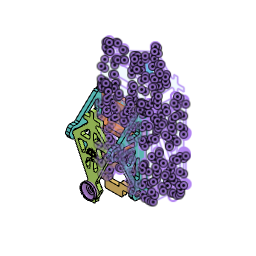
Katapult (Autodesk Fusion 360 design; units mm, degrees)
Autodesk Fusion 360 part; units mm, degrees
note: some values were not read from the file. Set by a fixed rule: which sketch regions a step uses.
(part 1 of 4)
sketch "Boden" plane through (0, 0, 0) normal (0, 1, 0) x (1, 0, 0)
  spline S0 degree 2 poles (146.3852, 44) (139.1926, 44) (132, 44) knots 58.903837 58.903837 58.903837 73.289058 73.289058 73.289058
  spline S1 degree 2 poles (132, 60) (138.2551, 60) (144.5102, 60) knots 21.966793 21.966793 21.966793 36.979059 36.979059 36.979059
  arc A0 (114.6662, 47.5529) -> (117.6148, 44) centre (117.6148, 47) ccw
  spline S2 degree 2 poles (119.4898, 60) (125.7449, 60) (132, 60) knots 109.599057 109.599057 109.599057 124.611322 124.611322 124.611322
  spline S3 degree 2 poles (147.4588, 57.5529) (148.3963, 52.5529) (149.3338, 47.5529) knots 41.135404 41.135404 41.135404 53.635404 53.635404 53.635404
  spline S4 degree 2 poles (132, 44) (124.8074, 44) (117.6148, 44) knots 73.289058 73.289058 73.289058 87.674279 87.674279 87.674279
  arc A1 (119.4898, 60) -> (116.5412, 57.5529) centre (119.4898, 57) ccw
  spline S5 degree 2 poles (114.6662, 47.5529) (115.6037, 52.5529) (116.5412, 57.5529) knots 92.942712 92.942712 92.942712 105.442712 105.442712 105.442712
  arc A2 (147.4588, 57.5529) -> (144.5102, 60) centre (144.5102, 57) ccw
  arc A3 (146.3852, 44) -> (149.3338, 47.5529) centre (146.3852, 47) ccw
  line L0 (157, 37.5) -> (157, 72.5)
  line L1 (107, 72.5) -> (107, 37.5)
  line L2 (157, 22.5) -> (162, 22.5)
  line L3 (162, 22.5) -> (162, 37.5)
  line L4 (162, 37.5) -> (157, 37.5)
  line L5 (157, 22.5) -> (157, 4)
  line L6 (157, 4) -> (107, 4)
  line L7 (107, 4) -> (107, 22.5)
  line L8 (107, 22.5) -> (102, 22.5)
  line L9 (102, 22.5) -> (102, 37.5)
  line L10 (102, 37.5) -> (107, 37.5)
  line L11 (107, 72.5) -> (102, 72.5)
  line L12 (102, 72.5) -> (102, 90.5)
  line L13 (157, 72.5) -> (162, 72.5)
  line L14 (162, 72.5) -> (162, 90.5)
  line L15 (120.5, 34) -> (143.5, 34)
  line L16 (143.5, 34) -> (143.5, 39)
  line L17 (143.5, 39) -> (120.5, 39)
  line L18 (120.5, 39) -> (120.5, 34)
  line L19 (102, 90.5) -> (107, 90.5)
  line L20 (107, 90.5) -> (107, 92)
  line L21 (157, 92) -> (157, 90.5)
  line L22 (157, 90.5) -> (162, 90.5)
  line L23 (107, 104) -> (107, 92)
  line L24 (107, 104) -> (117, 104)
  line L25 (117, 104) -> (117, 94)
  line L26 (117, 94) -> (132, 84.0491)
  line L27 (132, 84.0491) -> (147, 94)
  line L28 (147, 94) -> (147, 104)
  line L29 (147, 104) -> (156.9838, 104)
  line L30 (156.9838, 104) -> (157, 92)
  line L31 (114, 10) -> (127, 10)
  line L32 (127, 10) -> (114, 20)
  line L33 (114, 20) -> (114, 10)
  line L34 (150, 10) -> (137, 10)
  line L35 (137, 10) -> (150, 20)
  line L36 (150, 20) -> (150, 10)
  line L37 (127, 29) -> (127, 15)
  line L38 (127, 15) -> (109, 29)
  line L39 (109, 29) -> (127, 29)
  line L40 (137, 15) -> (155, 29)
  line L41 (155, 29) -> (137, 29)
  line L42 (137, 29) -> (137, 15)
  line L43 (129, 75) -> (129, 65)
  line L44 (129, 65) -> (115, 65)
  line L45 (115, 65) -> (115, 85)
  line L46 (115, 85) -> (129, 75)
  line L47 (135, 65) -> (149, 65)
  line L48 (149, 65) -> (149, 85)
  line L49 (149, 85) -> (135, 75)
  line L50 (135, 75) -> (135, 65)
  constraint horizontal L2
  constraint perpendicular L2 L3
  constraint perpendicular L2 L5
  constraint perpendicular L5 L6
  constraint parallel L6 L8
  constraint perpendicular L8 L9
  constraint perpendicular L1 L11
  constraint perpendicular L11 L12
  constraint perpendicular L0 L13
  constraint perpendicular L13 L14
  constraint horizontal L15
  constraint vertical L16
  constraint horizontal L17
  constraint vertical L18
  constraint perpendicular L12 L19
  constraint horizontal L22
  constraint perpendicular L23 L24
  constraint perpendicular L24 L25
  constraint parallel L25 L28
  constraint perpendicular L28 L29
  constraint horizontal L13
  constraint perpendicular L7 L31
  constraint perpendicular L31 L33
  constraint horizontal L34
  constraint perpendicular L34 L36
  constraint vertical L37
  constraint perpendicular L37 L39
  constraint horizontal L41
  constraint perpendicular L41 L42
  constraint parallel L42 L43
  constraint perpendicular L43 L44
  constraint perpendicular L44 L45
  constraint perpendicular L43 L47
  constraint perpendicular L47 L48
  constraint perpendicular L47 L50
sketch "Halter" plane through (0, 0, 0) normal (0, 1, 0) x (1, 0, 0)
  spline S0 degree 2 poles (99.3634, 51.0396) (99.5525, 51.4619) (99.5525, 51.9341) knots -102.762151 -102.762151 -102.762151 -101.834856 -101.834856 -101.834856 weights 1 0.973249 1
  spline S1 degree 2 poles (98.2087, 103.4619) (98.2087, 104.4619) (97.3128, 104.4619) knots -41.403496 -41.403496 -41.403496 -39.8327 -39.8327 -39.8327 weights 1 0.707107 1
  line L0 (83.4263, 70.9619) -> (83.4263, 63.4619)
  spline S2 degree 2 poles (93.7291, 43.4619) (93.7291, 42.4619) (94.6251, 42.4619) knots -116.78571 -116.78571 -116.78571 -115.214913 -115.214913 -115.214913 weights 1 0.707107 1
  spline S3 degree 2 poles (90.5935, 61.4619) (92.3853, 61.4619) (92.3853, 59.4619) knots -136.264428 -136.264428 -136.264428 -133.122835 -133.122835 -133.122835 weights 1 0.707107 1
  line L1 (83.4263, 75.9619) -> (83.4263, 70.9619)
  spline S4 degree 2 poles (83.4263, 63.4619) (83.4263, 61.4619) (85.2181, 61.4619) knots -145.40602 -145.40602 -145.40602 -142.264428 -142.264428 -142.264428 weights 1 0.707107 1
  spline S5 degree 2 poles (92.5745, 95.8842) (92.3853, 95.4619) (92.3853, 94.9898) knots -27.379937 -27.379937 -27.379937 -26.452642 -26.452642 -26.452642 weights 1 0.973249 1
  line L2 (94.6251, 42.4619) -> (97.3128, 42.4619)
  line L3 (93.7291, 103.4619) -> (93.7291, 98.4619)
  line L4 (97.7607, 66.4619) -> (94.1771, 66.4619)
  spline S6 degree 2 poles (92.3853, 51.9341) (92.3853, 51.4619) (92.5745, 51.0396) knots -125.594971 -125.594971 -125.594971 -124.667676 -124.667676 -124.667676 weights 1 0.973249 1
  line L5 (99.5525, 51.9341) -> (99.5525, 64.4619)
  spline S7 degree 2 poles (97.7607, 80.4619) (99.5525, 80.4619) (99.5525, 82.4619) knots -65.882214 -65.882214 -65.882214 -62.740621 -62.740621 -62.740621 weights 1 0.707107 1
  line L6 (93.7291, 48.4619) -> (93.7291, 43.4619)
  line L7 (99.5525, 82.4619) -> (99.5525, 94.9898)
  line L8 (94.1771, 80.4619) -> (97.7607, 80.4619)
  line L9 (94.1771, 73.4619) -> (94.1771, 80.4619)
  line L10 (93.7291, 98.4619) -> (92.5745, 95.8842)
  line L11 (94.1771, 66.4619) -> (94.1771, 73.4619)
  line L12 (98.2087, 98.4619) -> (98.2087, 103.4619)
  line L13 (92.3853, 59.4619) -> (92.3853, 51.9341)
  spline S8 degree 2 poles (92.3853, 87.4619) (92.3853, 85.4619) (90.5935, 85.4619) knots -18.924778 -18.924778 -18.924778 -15.783185 -15.783185 -15.783185 weights 1 0.707107 1
  line L14 (85.2181, 61.4619) -> (90.5935, 61.4619)
  spline S9 degree 2 poles (99.5525, 94.9898) (99.5525, 95.4619) (99.3634, 95.8842) knots -50.212757 -50.212757 -50.212757 -49.285462 -49.285462 -49.285462 weights 1 0.973249 1
  spline S10 degree 2 poles (99.5525, 64.4619) (99.5525, 66.4619) (97.7607, 66.4619) knots -89.306992 -89.306992 -89.306992 -86.165399 -86.165399 -86.165399 weights 1 0.707107 1
  line L15 (98.2087, 43.4619) -> (98.2087, 48.4619)
  line L16 (92.3853, 94.9898) -> (92.3853, 87.4619)
  spline S11 degree 2 poles (94.6251, 104.4619) (93.7291, 104.4619) (93.7291, 103.4619) knots -36.8327 -36.8327 -36.8327 -35.261903 -35.261903 -35.261903 weights 1 0.707107 1
  line L17 (92.5745, 51.0396) -> (93.7291, 48.4619)
  line L18 (83.4263, 83.4619) -> (83.4263, 75.9619)
  spline S12 degree 2 poles (85.2181, 85.4619) (83.4263, 85.4619) (83.4263, 83.4619) knots -9.783185 -9.783185 -9.783185 -6.641593 -6.641593 -6.641593 weights 1 0.707107 1
  line L19 (97.3128, 104.4619) -> (94.6251, 104.4619)
  line L20 (90.5935, 85.4619) -> (85.2181, 85.4619)
  spline S13 degree 2 poles (97.3128, 42.4619) (98.2087, 42.4619) (98.2087, 43.4619) knots -112.214913 -112.214913 -112.214913 -110.644117 -110.644117 -110.644117 weights 1 0.707107 1
  line L21 (99.3634, 95.8842) -> (98.2087, 98.4619)
  line L22 (98.2087, 48.4619) -> (99.3634, 51.0396)
sketch "Seiten" plane through (0, 0, 0) normal (0, 1, 0) x (1, 0, 0)
  spline S0 degree 2 poles (8, 106) (5.5, 106) (3, 106) knots -333.29607 -333.29607 -333.29607 -328.29607 -328.29607 -328.29607
  line L0 (0, 42) -> (0, 41)
  line L1 (11.4183, 106) -> (8, 106)
  arc A0 (1, 43) -> (3, 45) centre (1, 45) ccw
  line L2 (38.5159, 82.0817) -> (14.1539, 104.9183)
  arc A1 (14.1539, 104.9183) -> (11.4183, 106) centre (11.4183, 102) ccw
  line L3 (3, 66) -> (3, 45)
  arc A2 (1, 43) -> (0, 42) centre (1, 42) ccw
  arc A3 (3, 66) -> (1, 68) centre (1, 66) ccw
  arc A4 (0, 69) -> (1, 68) centre (1, 69) ccw
  line L4 (0, 103) -> (0, 69)
  arc A5 (3, 106) -> (0, 103) centre (3, 103) ccw
  arc A6 (49.4848, 79) -> (46.0207, 81) centre (46.0207, 77) ccw
  arc A7 (38.5159, 82.0817) -> (41.2515, 81) centre (41.2515, 85) ccw
  line L5 (42.2092, 66) -> (46.0207, 66)
  arc A8 (18.9309, 21.8917) -> (19.0866, 18.1897) centre (22.5507, 20.1897) ccw
  circle A9 centre (14, 13) radius 3.5355
  line L6 (18.9309, 21.8917) -> (38.5894, 63.702)
  arc A10 (20.9282, 11) -> (20.9282, 15) centre (17.4641, 13) ccw
  arc A11 (42.2092, 66) -> (38.5894, 63.702) centre (42.2092, 62) ccw
  line L7 (20.9282, 15) -> (19.0866, 18.1897)
  line L8 (51.5056, 75.5) -> (49.4848, 79)
  circle A12 centre (44, 73.5) radius 3.5355
  line L9 (49.4848, 68) -> (51.5056, 71.5)
  line L10 (9.9585, 6) -> (15.7321, 6)
  arc A13 (51.5056, 71.5) -> (51.5056, 75.5) centre (48.0415, 73.5) ccw
  arc A14 (0, 9) -> (3, 6) centre (3, 9) ccw
  line L11 (19.1962, 8) -> (20.9282, 11)
  arc A15 (15.7321, 6) -> (19.1962, 8) centre (15.7321, 10) ccw
  line L12 (46.0207, 81) -> (41.2515, 81)
  line L13 (0, 41) -> (0, 9)
  line L14 (3, 6) -> (9.9585, 6)
  arc A16 (46.0207, 66) -> (49.4848, 68) centre (46.0207, 70) ccw
  line L15 (18.5, 71) -> (33.5, 71)
  line L16 (33.5, 71) -> (33.5, 76)
  line L17 (33.5, 76) -> (18.5, 76)
  line L18 (18.5, 76) -> (18.5, 71)
  line L19 (3, 72.5) -> (8, 72.5)
  line L20 (8, 72.5) -> (8, 87.5)
  line L21 (8, 87.5) -> (3, 87.5)
  line L22 (3, 87.5) -> (3, 72.5)
  line L23 (3, 19.5) -> (8, 19.5)
  line L24 (8, 19.5) -> (8, 37.5)
  line L25 (8, 37.5) -> (3, 37.5)
  line L26 (3, 37.5) -> (3, 19.5)
  line L27 (12, 20) -> (12, 62)
  line L28 (12, 62) -> (23, 43)
  line L29 (23, 43) -> (12, 20)
  line L30 (34, 66) -> (26, 48)
  line L31 (26, 48) -> (15.5, 66)
  line L32 (15.5, 66) -> (34, 66)
  line L33 (12, 81) -> (32.5, 81)
  line L34 (32.5, 81) -> (12, 100)
  line L35 (12, 100) -> (12, 81)
  dimension "d27" = 15
  constraint horizontal L15
  constraint vertical L16
  constraint horizontal L17
  constraint vertical L18
  constraint horizontal L19
  constraint vertical L20
  constraint horizontal L21
  constraint vertical L22
  constraint horizontal L23
  constraint vertical L24
  constraint horizontal L25
  constraint vertical L26
  constraint vertical L27
  constraint horizontal L32
  constraint horizontal L33
  constraint perpendicular L33 L35
  measures "d27" distance of L16.end L17.end
sketch "Hebel" plane through (0, 0, 0) normal (0, 1, 0) x (1, 0, 0)
  line L0 (73.128, 41.6803) -> (76.7542, 51.7057)
  spline S0 degree 2 poles (42, 34) (51.4199, 25.1097) (60.8397, 16.2193) (61.8269, 15.2877) (61.3256, 14.0262) (60.8244, 12.7648) (59.467, 12.7648) (58.2335, 12.7648) (57, 12.7648) (56, 12.7648) (56, 11.7648) (56, 10.2648) (56, 8.7648) (56, 7.7648) (57, 7.7648) (59.75, 7.7648) (62.5, 7.7648) (64.5, 7.7648) (64.5, 5.7648) (64.5, 3.0148) (64.5, 0.2648) (64.5, -0.7352) (65.5, -0.7352) (67, -0.7352) (68.5, -0.7352) (69.5, -0.7352) (69.5, 0.2648) (69.5, 3.0148) (69.5, 5.7648) (69.5, 7.7648) (71.5, 7.7648) (74.25, 7.7648) (77, 7.7648) (78, 7.7648) (78, 8.7648) (78, 10.2648) (78, 11.7648) (78, 12.7648) (77, 12.7648) (75.7665, 12.7648) (74.533, 12.7648) (73.1756, 12.7648) (72.6744, 14.0262) (72.1731, 15.2877) (73.1603, 16.2193) (82.5801, 25.1097) (92, 34) knots -180.29335 -180.29335 -180.29335 -154.387975 -154.387975 -152.002869 -152.002869 -149.617763 -149.617763 -147.150765 -147.150765 -145.579969 -145.579969 -142.579969 -142.579969 -141.009172 -141.009172 -135.509172 -135.509172 -132.36758 -132.36758 -126.86758 -126.86758 -125.296783 -125.296783 -122.296783 -122.296783 -120.725987 -120.725987 -115.225987 -115.225987 -112.084394 -112.084394 -106.584394 -106.584394 -105.013598 -105.013598 -102.013598 -102.013598 -100.442802 -100.442802 -97.975804 -97.975804 -95.590698 -95.590698 -93.205592 -93.205592 -67.300216 -67.300216 -67.300216 weights 1 1 1 0.827432 1 0.827432 1 1 1 0.707107 1 1 1 0.707107 1 1 1 0.707107 1 1 1 0.707107 1 1 1 0.707107 1 1 1 0.707107 1 1 1 0.707107 1 1 1 0.707107 1 1 1 0.827432 1 0.827432 1 1 1
  arc A0 (83.3325, 39) -> (85.1436, 41.8486) centre (83.3325, 41) ccw
  arc A1 (75.1144, 61.8724) -> (75.0447, 63.4012) centre (73.2337, 62.5527) ccw
  line L1 (71.5, 34) -> (79.6823, 34)
  line L2 (81.055, 30.5455) -> (72.8727, 22.8232)
  line L3 (69.5, 24.2777) -> (69.5, 32)
  arc A2 (73.311, 67.1012) -> (69.5, 66.2526) centre (71.5, 66.2526) ccw
  line L4 (69.5, 66.2526) -> (69.5, 57.7595)
  arc A3 (80.446, 51.8741) -> (76.7542, 51.7057) centre (78.6349, 51.0255) ccw
  line L5 (80.446, 51.8741) -> (85.1436, 41.8486)
  arc A4 (61.1273, 22.8232) -> (64.5, 24.2777) centre (62.5, 24.2777) ccw
  line L6 (64.5, 24.2777) -> (64.5, 32)
  arc A5 (54.3177, 34) -> (52.945, 30.5455) centre (54.3177, 32) ccw
  line L7 (52.945, 30.5455) -> (61.1273, 22.8232)
  arc A6 (48.8564, 41.8486) -> (50.6675, 39) centre (50.6675, 41) ccw
  line L8 (50.6675, 39) -> (58.9913, 39)
  arc A7 (71.5, 34) -> (69.5, 32) centre (71.5, 32) ccw
  line L9 (62.5, 34) -> (54.3177, 34)
  arc A8 (69.5, 24.2777) -> (72.8727, 22.8232) centre (71.5, 24.2777) ccw
  line L10 (73.3808, 57.0792) -> (75.1144, 61.8724)
  arc A9 (60.6192, 57.0792) -> (64.5, 57.7595) centre (62.5, 57.7595) ccw
  line L11 (60.6192, 57.0792) -> (58.8856, 61.8724)
  line L12 (83.3325, 39) -> (75.0087, 39)
  arc A10 (73.128, 41.6803) -> (75.0087, 39) centre (75.0087, 41) ccw
  arc A11 (69.5, 57.7595) -> (73.3808, 57.0792) centre (71.5, 57.7595) ccw
  arc A12 (64.5, 32) -> (62.5, 34) centre (62.5, 32) ccw
  line L13 (60.872, 41.6803) -> (57.2458, 51.7057)
  arc A13 (58.9913, 39) -> (60.872, 41.6803) centre (58.9913, 41) ccw
  line L14 (58.9553, 63.4012) -> (60.689, 67.1012)
  arc A14 (64.5, 66.2526) -> (60.689, 67.1012) centre (62.5, 66.2526) ccw
  line L15 (64.5, 66.2526) -> (64.5, 57.7595)
  arc A15 (57.2458, 51.7057) -> (53.554, 51.8741) centre (55.3651, 51.0255) ccw
  arc A16 (81.055, 30.5455) -> (79.6823, 34) centre (79.6823, 32) ccw
  arc A17 (58.9553, 63.4012) -> (58.8856, 61.8724) centre (60.7663, 62.5527) ccw
  line L16 (53.554, 51.8741) -> (48.8564, 41.8486)
  line L17 (75.0447, 63.4012) -> (73.311, 67.1012)
  spline S1 degree 2 poles (98, 38) (98, 39) (97, 39) (94.5, 39) (92, 39) knots -57.72942 -57.72942 -57.72942 -56.158624 -56.158624 -51.158624 -51.158624 -51.158624 weights 1 0.707107 1 1 1
  spline S2 degree 2 poles (92, 34) (94.5, 34) (97, 34) (98, 34) (98, 35) knots -67.300216 -67.300216 -67.300216 -62.300216 -62.300216 -60.72942 -60.72942 -60.72942 weights 1 1 1 0.707107 1
  line L18 (98, 35) -> (98, 38)
  line L19 (36, 37.9531) -> (36, 38)
  spline S3 degree 2 poles (36, 35) (36, 34) (37, 34) (39.5, 34) (42, 34) knots -186.864147 -186.864147 -186.864147 -185.29335 -185.29335 -180.29335 -180.29335 -180.29335 weights 1 0.707107 1 1 1
  spline S4 degree 2 poles (42, 39) (39.5, 39) (37, 39) (36, 39) (36, 38) (36, 37.9766) (36, 37.9531) knots -196.434943 -196.434943 -196.434943 -191.434943 -191.434943 -189.864147 -189.864147 -189.817295 -189.817295 -189.817295 weights 1 1 1 0.707107 1 1 1
  line L20 (36, 35) -> (36, 37.9531)
  circle A18 centre (67, 90.2648) radius 0.375
  line L21 (72.1962, 102.2483) -> (72.1962, 103.0296)
  line L22 (69.4512, 105.0296) -> (70.1962, 105.0296)
  line L23 (67, 105.0296) -> (62, 105.0296)
  line L24 (62, 105.0296) -> (62, 100)
  line L25 (62, 100) -> (56.5, 90)
  line L26 (56.5, 90) -> (62, 81)
  line L27 (62, 81) -> (42, 39)
  line L28 (67, 105.0296) -> (72, 105.0296)
  line L29 (72, 105.0296) -> (72, 100)
  line L30 (72, 100) -> (77.5, 90)
  line L31 (77.5, 90) -> (72, 81)
  line L32 (72, 81) -> (92, 39)
  dimension "d48" = 0.75
  constraint coincident L19.end S4
  constraint vertical L19
  constraint vertical L21
  constraint perpendicular L21 L22
  constraint horizontal L23
  constraint perpendicular L23 L24
  constraint perpendicular L23 L29
  measures "d48" diameter of A18
sketch "Quer" plane through (0, 0, 0) normal (0, 1, 0) x (1, 0, 0)
  line L0 (163.6644, 44.088) -> (163.6644, 30.588)
  line L1 (163.6644, 80.588) -> (163.6644, 67.088)
  line L2 (163.6644, 67.088) -> (158.6644, 67.088)
  line L3 (158.6644, 44.088) -> (163.6644, 44.088)
  line L4 (163.6644, 30.588) -> (174.1644, 30.588)
  line L5 (174.1644, 80.588) -> (163.6644, 80.588)
  line L6 (174.1644, 85.588) -> (174.1644, 80.588)
  arc A0 (175.8002, 69.9888) -> (174.6644, 67.6383) centre (177.6644, 67.6383) ccw
  line L7 (189.1644, 85.588) -> (174.1644, 85.588)
  line L8 (189.1644, 80.588) -> (189.1644, 85.588)
  line L9 (174.6644, 55.588) -> (174.6644, 67.6383)
  line L10 (174.1644, 30.588) -> (174.1644, 25.588)
  line L11 (189.1644, 25.588) -> (189.1644, 30.588)
  line L12 (174.6644, 43.5376) -> (174.6644, 55.588)
  arc A1 (174.6644, 43.5376) -> (175.8002, 41.1871) centre (177.6644, 43.5376) ccw
  line L13 (174.1644, 25.588) -> (189.1644, 25.588)
  line L14 (158.6644, 67.088) -> (158.6644, 44.088)
  line L15 (189.1644, 30.588) -> (191, 30.588)
  line L16 (191, 30.588) -> (191, 32)
  line L17 (191, 32) -> (175.8002, 41.1871)
  line L18 (189.1644, 80.588) -> (191, 80.588)
  line L19 (191, 80.588) -> (191, 79)
  line L20 (191, 79) -> (175.8002, 69.9888)
  constraint perpendicular L11 L15
  constraint perpendicular L15 L16
  constraint perpendicular L16 L18
  constraint perpendicular L15 L19
sketch "makerhafen-logo" plane through (78.9239, 0, 23.4593) normal (0, 1, 0) x (1, 0, 0)
  line L0 (3.0435, 0.3482) -> (3.0389, 0.4531)
  line L1 (3.0389, 0.4531) -> (3.0716, 0.553)
  line L2 (2.5336, 2.4375) -> (2.6594, 2.4375)
  line L3 (3.8976, 2.125) -> (3.8976, 2.0272)
  line L4 (3.3321, 2.1809) -> (3.3321, 2.0276)
  line L5 (1.114, 2.2681) -> (1.2274, 2.4375)
  line L6 (1.2274, 2.4375) -> (1.3404, 2.4375)
  line L7 (1.3404, 2.4375) -> (1.237, 2.2876)
  line L8 (1.237, 2.2876) -> (1.3653, 2.0276)
  line L9 (3.8536, 1.161) -> (3.855, 1.1648)
  line L10 (3.8701, 1.2062) -> (3.8445, 1.2134)
  line L11 (3.773, 1.2543) -> (3.7021, 1.3317)
  line L12 (0, 2.4375) -> (0.1643, 2.4375)
  line L13 (0.1643, 2.4375) -> (0.2237, 2.2199)
  line L14 (0.2237, 2.2199) -> (0.2804, 2.4375)
  line L15 (0.2804, 2.4375) -> (0.4453, 2.4375)
  line L16 (0.0938, 2.0276) -> (0, 2.0276)
  line L17 (0, 2.0276) -> (0, 2.4375)
  line L18 (3.8445, 1.2134) -> (3.773, 1.2543)
  line L19 (2.4219, 0.1221) -> (2.4498, 0.0447)
  line L20 (2.4498, 0.0447) -> (2.4525, 0.0182)
  line L21 (2.4525, 0.0182) -> (2.4564, 0.0189)
  line L22 (3.7483, 1.1867) -> (3.8294, 1.172)
  line L23 (3.855, 1.1648) -> (3.8688, 1.2024)
  line L24 (3.6442, 1.1731) -> (3.7483, 1.1867)
  line L25 (3.6571, 1.5112) -> (3.6617, 1.5374)
  line L26 (3.5413, 0.6742) -> (3.4882, 0.7372)
  line L27 (3.0719, 0.2709) -> (3.0435, 0.3482)
  line L28 (3.087, 0.2489) -> (3.0719, 0.2709)
  line L29 (3.4414, 0.6821) -> (3.5126, 0.6406)
  line L30 (3.4481, 0.8343) -> (3.4449, 0.9392)
  line L31 (3.1608, 0.654) -> (3.2349, 0.6899)
  line L32 (3.0389, 0.4531) -> (3.0716, 0.553)
  line L33 (2.3853, 3.8451) -> (2.3988, 3.8779)
  line L34 (2.3988, 3.8779) -> (2.4006, 3.8841)
  line L35 (1.6118, 0.4999) -> (1.4882, 0.5595)
  line L36 (3.2349, 0.6899) -> (3.3389, 0.7049)
  line L37 (3.5126, 0.6406) -> (3.5317, 0.622)
  line L38 (3.5603, 0.6555) -> (3.5629, 0.6586)
  line L39 (3.5516, 1.1236) -> (3.6442, 1.1731)
  line L40 (3.4676, 1.0185) -> (3.4809, 1.0414)
  line L41 (3.3389, 0.7049) -> (3.4414, 0.6821)
  line L42 (3.1404, 0.6368) -> (3.1608, 0.654)
  line L43 (3.4882, 0.7372) -> (3.4481, 0.8343)
  line L44 (1.7416, 0.4524) -> (1.6118, 0.4999)
  line L45 (3.12, 0.6197) -> (3.1404, 0.6368)
  line L46 (3.0716, 0.553) -> (3.12, 0.6197)
  line L47 (3.5629, 0.6586) -> (3.5413, 0.6742)
  line L48 (3.0435, 0.3482) -> (3.0389, 0.4531)
  line L49 (3.4809, 1.0414) -> (3.4942, 1.0645)
  line L50 (3.5343, 0.625) -> (3.5603, 0.6555)
  line L51 (3.5317, 0.622) -> (3.5343, 0.625)
  line L52 (2.2074, 2.3253) -> (2.2071, 2.3169)
  line L53 (2.2071, 2.3169) -> (2.2072, 2.3115)
  line L54 (2.2072, 2.3115) -> (2.1951, 2.2592)
  line L55 (3.7128, 2.343) -> (3.7128, 2.2835)
  line L56 (2.1927, 2.2544) -> (2.1903, 2.2499)
  line L57 (2.1951, 2.2592) -> (2.1927, 2.2544)
  line L58 (1.4324, 0.369) -> (1.5352, 0.3905)
  line L59 (0.9862, 0.7052) -> (1.0901, 0.6902)
  line L60 (2.358, 0.2054) -> (2.4219, 0.1221)
  line L61 (2.4998, 0.0265) -> (2.4932, 0.0523)
  line L62 (0.7626, 0.6593) -> (0.7651, 0.6562)
  line L63 (1.9666, 0.2054) -> (2.0558, 0.2607)
  line L64 (0.3556, 1.8261) -> (0.3556, 1.8201)
  line L65 (1.6171, 0.382) -> (1.6422, 0.3729)
  line L66 (1.3437, 0.3126) -> (1.4324, 0.369)
  line L67 (2.3434, 1.1709) -> (2.3441, 1.1666)
  line L68 (2.3441, 1.1666) -> (2.3953, 0.9132)
  line L69 (2.3953, 0.9132) -> (2.3955, 0.9124)
  line L70 (2.3955, 0.9124) -> (2.3964, 0.9052)
  line L71 (1.6422, 0.3729) -> (1.6672, 0.3638)
  line L72 (2.0687, 1.6326) -> (2.0687, 1.604)
  line L73 (2.0687, 1.604) -> (2.0684, 1.6011)
  line L74 (2.0684, 1.6011) -> (2.0676, 1.596)
  line L75 (3.5126, 0.6406) -> (3.5317, 0.622)
  line L76 (3.5317, 0.622) -> (3.5343, 0.625)
  line L77 (2.5894, 0.3175) -> (2.6576, 0.3637)
  line L78 (1.0901, 0.6902) -> (1.1642, 0.6542)
  line L79 (2.9769, 2.1084) -> (2.8671, 2.1084)
  line L80 (2.0236, 2.2719) -> (2.027, 2.2717)
  line L81 (1.8443, 2.4375) -> (2.058, 2.4375)
  line L82 (2.4525, 0.0182) -> (2.4564, 0.0189)
  line L83 (2.4498, 0.0447) -> (2.4525, 0.0182)
  line L84 (2.4958, 0.0258) -> (2.4998, 0.0265)
  line L85 (2.3964, 0.9052) -> (2.3964, 0.9028)
  line L86 (2.3964, 0.9028) -> (2.4026, 0.9061)
  line L87 (2.4026, 0.9061) -> (2.4176, 0.9228)
  line L88 (2.4176, 0.9228) -> (2.438, 0.9563)
  line L89 (0.8373, 0.7378) -> (0.7842, 0.6749)
  line L90 (0.6599, 1.5643) -> (0.6646, 1.5381)
  line L91 (0.3556, 1.8066) -> (0.3556, 1.8021)
  line L92 (2.8925, 0.3688) -> (2.9811, 0.3122)
  line L93 (0.7651, 0.6562) -> (0.7907, 0.6255)
  line L94 (3.0488, 0.2268) -> (3.0834, 0.2468)
  line L95 (1.7354, 0.3175) -> (1.8003, 0.2349)
  line L96 (3.3802, 1.8021) -> (3.3802, 1.8081)
  line L97 (0.7933, 0.6225) -> (0.8124, 0.6411)
  line L98 (0.8124, 0.6411) -> (0.8836, 0.6825)
  line L99 (2.4564, 0.0189) -> (2.4958, 0.0258)
  line L100 (3.0337, 0.2489) -> (3.0453, 0.2249)
  line L101 (1.8249, 0.0265) -> (1.8288, 0.0258)
  line L102 (2.5245, 0.2349) -> (2.5894, 0.3175)
  line L103 (2.4932, 0.0523) -> (2.4928, 0.1347)
  line L104 (1.2795, 0.2252) -> (1.291, 0.2492)
  line L105 (3.5343, 0.625) -> (3.5603, 0.6555)
  line L106 (3.5603, 0.6555) -> (3.5629, 0.6586)
  line L107 (3.5629, 0.6586) -> (3.5413, 0.6742)
  line L108 (2.0676, 1.596) -> (2.0534, 1.5462)
  line L109 (2.0534, 1.5462) -> (2.0514, 1.5414)
  line L110 (2.0514, 1.5414) -> (2.0497, 1.5367)
  line L111 (2.9811, 0.3122) -> (3.0337, 0.2489)
  line L112 (0.3556, 1.783) -> (0.3556, 1.7787)
  line L113 (1.2813, 0.3485) -> (1.2528, 0.2712)
  line L114 (2.4928, 0.1347) -> (2.5245, 0.2349)
  line L115 (3.0716, 0.553) -> (3.12, 0.6197)
  line L116 (3.12, 0.6197) -> (3.1404, 0.6368)
  line L117 (3.1404, 0.6368) -> (3.1608, 0.654)
  line L118 (2.3255, 1.1962) -> (2.3376, 1.1836)
  line L119 (2.3376, 1.1836) -> (2.3434, 1.1709)
  line L120 (1.9026, 0.1221) -> (1.9666, 0.2054)
  line L121 (2.7077, 0.3819) -> (2.7896, 0.3903)
  line L122 (1.2859, 0.4534) -> (1.2813, 0.3485)
  line L123 (1.2378, 0.2492) -> (1.2412, 0.2471)
  line L124 (2.6827, 0.3728) -> (2.7077, 0.3819)
  line L125 (2.6576, 0.3637) -> (2.6827, 0.3728)
  line L126 (1.8315, 0.0523) -> (1.8249, 0.0265)
  line L127 (2.438, 0.9563) -> (2.4559, 0.9966)
  line L128 (2.4559, 0.9966) -> (2.4665, 1.0268)
  line L129 (1.1846, 0.637) -> (1.2049, 0.62)
  line L130 (1.8003, 0.2349) -> (1.8318, 0.1347)
  line L131 (2.1356, 0.2808) -> (2.1623, 0.2808)
  line L132 (1.2049, 0.62) -> (1.2532, 0.5532)
  line L133 (1.8721, 0.0182) -> (1.8747, 0.0447)
  line L134 (1.9786, 1.3712) -> (1.9629, 1.3493)
  line L135 (1.9629, 1.3493) -> (1.9461, 1.33)
  line L136 (1.9461, 1.33) -> (1.9287, 1.3096)
  line L137 (0.8776, 0.8348) -> (0.8373, 0.7378)
  line L138 (2.0385, 1.5022) -> (2.0354, 1.4931)
  line L139 (2.0354, 1.4931) -> (2.0344, 1.49)
  line L140 (2.0344, 1.49) -> (2.031, 1.4804)
  line L141 (2.2687, 0.2607) -> (2.358, 0.2054)
  line L142 (3.1608, 0.654) -> (3.2349, 0.6899)
  line L143 (3.2349, 0.6899) -> (3.3389, 0.7049)
  line L144 (3.3389, 0.7049) -> (3.4414, 0.6821)
  line L145 (3.4414, 0.6821) -> (3.5126, 0.6406)
  line L146 (2.031, 1.4804) -> (1.9884, 1.3877)
  line L147 (1.9884, 1.3877) -> (1.9832, 1.3789)
  line L148 (1.9832, 1.3789) -> (1.9786, 1.3712)
  line L149 (1.2759, 0.2272) -> (1.2795, 0.2252)
  line L150 (2.7896, 0.3903) -> (2.8925, 0.3688)
  line L151 (0.845, 1.042) -> (0.8583, 1.019)
  line L152 (3.0834, 0.2468) -> (3.087, 0.2489)
  line L153 (1.8681, 0.0189) -> (1.8721, 0.0182)
  line L154 (2.1623, 0.2808) -> (2.1889, 0.2808)
  line L155 (2.0497, 1.5367) -> (2.0449, 1.5225)
  line L156 (2.0449, 1.5225) -> (2.0413, 1.5112)
  line L157 (2.0413, 1.5112) -> (2.0385, 1.5022)
  line L158 (4.0936, 2.2258) -> (4.0936, 2.0278)
  line L159 (2.058, 2.4375) -> (2.0737, 2.4375)
  line L160 (0.4964, 1.1729) -> (0.5775, 1.1875)
  line L161 (0.845, 1.042) -> (0.8583, 1.019)
  line L162 (0.6631, 1.4297) -> (0.6239, 1.3323)
  line L163 (0.5528, 1.2549) -> (0.4813, 1.214)
  line L164 (0.7651, 0.6562) -> (0.7907, 0.6255)
  line L165 (1.97, 2.0276) -> (1.8443, 2.0276)
  line L166 (1.8443, 2.0276) -> (1.8443, 2.4375)
  line L167 (1.7507, 2.343) -> (1.5659, 2.343)
  line L168 (1.5659, 2.343) -> (1.5659, 2.2835)
  line L169 (0.4722, 1.1619) -> (0.4964, 1.1729)
  line L170 (0.7743, 1.1242) -> (0.8317, 1.0651)
  line L171 (0.4813, 1.214) -> (0.4557, 1.2069)
  line L172 (0.7933, 0.6225) -> (0.8124, 0.6411)
  line L173 (3.4481, 0.8343) -> (3.4449, 0.9392)
  line L174 (3.4449, 0.9392) -> (3.4676, 1.0185)
  line L175 (3.4676, 1.0185) -> (3.4809, 1.0414)
  line L176 (0.5564, 1.7179) -> (0.6264, 1.6395)
  line L177 (0.3822, 1.7807) -> (0.4633, 1.7665)
  line L178 (0.8124, 0.6411) -> (0.8836, 0.6825)
  line L179 (2.1889, 0.2808) -> (2.2687, 0.2607)
  line L180 (2.2687, 0.2607) -> (2.358, 0.2054)
  line L181 (2.358, 0.2054) -> (2.4219, 0.1221)
  line L182 (0.7907, 0.6255) -> (0.7933, 0.6225)
  line L183 (1.5631, 3.3276) -> (1.5675, 3.3102)
  line L184 (1.5675, 3.3102) -> (1.5796, 3.2908)
  line L185 (1.5796, 3.2909) -> (1.5978, 3.2772)
  line L186 (1.5978, 3.2772) -> (1.6147, 3.2713)
  line L187 (1.6147, 3.2713) -> (1.6205, 3.2708)
  line L188 (0.7626, 0.6593) -> (0.7651, 0.6562)
  line L189 (3.5413, 0.6742) -> (3.4882, 0.7372)
  line L190 (3.4882, 0.7372) -> (3.4481, 0.8343)
  line L191 (0.6816, 1.1738) -> (0.7743, 1.1242)
  line L192 (0.6691, 1.5119) -> (0.6631, 1.4297)
  line L193 (0.9862, 0.7052) -> (1.0901, 0.6902)
  line L194 (2.3927, 4.0582) -> (2.3613, 4.1039)
  line L195 (2.3613, 4.1039) -> (2.3176, 4.138)
  line L196 (2.3176, 4.138) -> (2.2782, 4.1549)
  line L197 (2.4109, 3.9939) -> (2.4092, 4.0038)
  line L198 (2.4092, 4.0038) -> (2.4072, 4.0177)
  line L199 (2.4072, 4.0177) -> (2.3927, 4.0582)
  line L200 (1.0901, 0.6902) -> (1.1642, 0.6542)
  line L201 (0.8317, 1.0651) -> (0.845, 1.042)
  line L202 (0.3556, 1.7787) -> (0.3822, 1.7807)
  line L203 (0.3556, 1.7962) -> (0.3556, 1.783)
  line L204 (0.8776, 0.8348) -> (0.8373, 0.7378)
  line L205 (0.4633, 1.7665) -> (0.5564, 1.7179)
  line L206 (0.8836, 0.6825) -> (0.9862, 0.7052)
  line L207 (0.8373, 0.7378) -> (0.7842, 0.6749)
  line L208 (1.1846, 0.637) -> (1.2049, 0.62)
  line L209 (0.8809, 0.9398) -> (0.8776, 0.8348)
  line L210 (1.6205, 3.2708) -> (1.6205, 3.4167)
  line L211 (1.6205, 3.4167) -> (1.6309, 3.4167)
  line L212 (0.5775, 1.1875) -> (0.6816, 1.1738)
  line L213 (0.6264, 1.6395) -> (0.6599, 1.5643)
  line L214 (0.8583, 1.019) -> (0.8809, 0.9398)
  line L215 (0.6239, 1.3323) -> (0.5528, 1.2549)
  line L216 (0.7842, 0.6749) -> (0.7626, 0.6593)
  line L217 (1.2049, 0.62) -> (1.2532, 0.5532)
  line L218 (1.1642, 0.6542) -> (1.1846, 0.637)
  line L219 (1.5659, 2.2835) -> (1.7153, 2.2835)
  line L220 (1.7153, 2.2835) -> (1.7153, 2.1926)
  line L221 (2.1623, 0.2808) -> (2.1889, 0.2808)
  line L222 (3.4809, 1.0414) -> (3.4942, 1.0645)
  line L223 (3.4942, 1.0645) -> (3.5516, 1.1236)
  line L224 (3.5516, 1.1236) -> (3.6442, 1.1731)
  line L225 (3.6442, 1.1731) -> (3.7483, 1.1867)
  line L226 (0.4706, 1.1656) -> (0.4722, 1.1619)
  line L227 (0.6646, 1.5381) -> (0.6691, 1.5119)
  line L228 (0.4557, 1.2069) -> (0.457, 1.2031)
  line L229 (1.4426, 2.4375) -> (1.7507, 2.4375)
  line L230 (1.97, 2.2719) -> (2.0237, 2.2719)
  line L231 (2.0695, 2.0276) -> (2.0096, 2.1839)
  line L232 (0.457, 1.2031) -> (0.4706, 1.1656)
  line L233 (1.5591, 0.9081) -> (1.3995, 1.0398)
  line L234 (1.0838, 1.8081) -> (1.0838, 1.8216)
  line L235 (1.1145, 2.1221) -> (1.1145, 2.0276)
  line L236 (1.3653, 2.0276) -> (1.2277, 2.0276)
  line L237 (0.6747, 2.1979) -> (0.741, 2.1979)
  line L238 (0.7631, 2.1084) -> (0.6533, 2.1084)
  line L239 (1.9446, 0.7459) -> (1.7422, 0.8087)
  line L240 (3.2844, 1.328) -> (3.3554, 1.5566)
  line L241 (2.1008, 0.5841) -> (2.1622, 0.584)
  line L242 (1.2532, 0.5532) -> (1.2859, 0.4534)
  line L243 (1.2859, 0.4534) -> (1.2813, 0.3485)
  line L244 (2.1622, 0.584) -> (2.2235, 0.584)
  line L245 (1.2629, 0.7116) -> (1.1625, 0.8028)
  line L246 (1.2679, 1.1993) -> (1.1685, 1.3824)
  line L247 (1.0838, 1.8021) -> (1.0838, 1.8081)
  line L248 (2.2782, 4.1549) -> (2.2645, 4.1577)
  line L249 (2.2645, 4.1577) -> (2.252, 4.1615)
  line L250 (2.252, 4.1615) -> (2.2126, 4.1664)
  line L251 (2.7647, 0.9081) -> (2.5815, 0.8087)
  line L252 (3.3802, 1.8261) -> (3.24, 1.8261)
  line L253 (1.3995, 1.0398) -> (1.2679, 1.1993)
  line L254 (2.4076, 0.6088) -> (2.6363, 0.6798)
  line L255 (3.2181, 1.5849) -> (3.1553, 1.3824)
  line L256 (3.8629, 1.7657) -> (3.944, 1.7798)
  line L257 (1.4882, 0.5595) -> (1.3717, 0.6302)
  line L258 (1.7507, 2.125) -> (1.7507, 2.0272)
  line L259 (1.2277, 2.0276) -> (1.157, 2.1824)
  line L260 (1.291, 0.2492) -> (1.3437, 0.3126)
  line L261 (1.3437, 0.3126) -> (1.4324, 0.369)
  line L262 (1.6013, 3.4743) -> (1.5814, 3.4609)
  line L263 (1.5814, 3.4609) -> (1.568, 3.441)
  line L264 (1.568, 3.441) -> (1.5632, 3.4228)
  line L265 (1.5632, 3.4228) -> (1.5632, 3.4167)
  line L266 (1.3717, 0.6302) -> (1.2629, 0.7116)
  line L267 (3.0559, 1.1993) -> (2.9242, 1.0398)
  line L268 (0.9192, 1.1285) -> (0.8596, 1.252)
  line L269 (1.7507, 2.0272) -> (1.4426, 2.0272)
  line L270 (1.8288, 0.0258) -> (1.8681, 0.0189)
  line L271 (3.9692, 1.8255) -> (3.965, 1.8253)
  line L272 (0.3288, 2.0279) -> (0.3288, 2.3204)
  line L273 (0.3288, 2.3204) -> (0.2531, 2.0276)
  line L274 (2.4344, 1.308) -> (2.401, 1.3634)
  line L275 (1.0713, 0.9032) -> (0.99, 1.0119)
  line L276 (3.944, 1.7798) -> (3.9705, 1.7778)
  line L277 (1.6257, 3.4792) -> (1.6195, 3.4792)
  line L278 (1.6195, 3.4792) -> (1.6013, 3.4743)
  line L279 (1.1523, 1.1212) -> (1.3011, 0.9409)
  line L280 (1.8747, 0.0447) -> (1.9026, 0.1221)
  line L281 (1.9026, 0.1221) -> (1.9666, 0.2054)
  line L282 (1.9666, 0.2054) -> (2.0558, 0.2607)
  line L283 (2.0558, 0.2607) -> (2.1356, 0.2808)
  line L284 (2.1356, 0.2808) -> (2.1623, 0.2808)
  line L285 (3.9692, 1.8255) -> (3.965, 1.8253)
  line L286 (1.2759, 0.2272) -> (1.2795, 0.2252)
  line L287 (1.2795, 0.2252) -> (1.291, 0.2492)
  line L288 (2.8432, 0.7921) -> (3.0234, 0.9408)
  line L289 (2.7644, 3.4742) -> (2.7462, 3.4792)
  line L290 (2.7462, 3.4792) -> (2.7402, 3.4792)
  line L291 (2.299, 3.1979) -> (2.082, 3.1979)
  line L292 (1.7354, 0.3175) -> (1.8003, 0.2349)
  line L293 (1.8003, 0.2349) -> (1.8318, 0.1347)
  line L294 (1.8318, 0.1347) -> (1.8315, 0.0523)
  line L295 (1.8315, 0.0523) -> (1.8249, 0.0265)
  line L296 (1.8249, 0.0265) -> (1.8288, 0.0258)
  line L297 (2.6363, 0.6798) -> (2.8432, 0.7921)
  line L298 (2.0364, 3.8065) -> (2.0398, 3.8017)
  line L299 (2.4607, 1.2504) -> (2.4553, 1.2652)
  line L300 (2.0929, 3.9887) -> (2.078, 4.0171)
  line L301 (2.078, 4.0171) -> (2.1081, 4.0203)
  line L302 (2.3055, 4.0203) -> (2.3355, 4.0171)
  line L303 (2.3355, 4.0171) -> (2.3206, 3.9887)
  line L304 (2.3206, 3.9887) -> (2.3487, 3.9768)
  line L305 (3.3554, 1.5566) -> (3.3802, 1.7407)
  line L306 (2.3251, 3.9181) -> (2.3433, 3.8922)
  line L307 (2.3433, 3.8922) -> (2.3141, 3.8845)
  line L308 (2.3141, 3.8845) -> (2.3252, 3.8542)
  line L309 (1.4426, 2.0272) -> (1.4426, 2.4375)
  line L310 (1.7507, 2.4375) -> (1.7507, 2.343)
  line L311 (1.1145, 2.0276) -> (0.9955, 2.0276)
  line L312 (0.9955, 2.0276) -> (0.9955, 2.4375)
  line L313 (1.9949, 3.9966) -> (1.9938, 3.9909)
  line L314 (1.9938, 3.9909) -> (1.9925, 3.9841)
  line L315 (1.9925, 3.9841) -> (1.9925, 3.9145)
  line L316 (2.1305, 4.0464) -> (2.1315, 4.0792)
  line L317 (2.1315, 4.0792) -> (2.1586, 4.065)
  line L318 (2.1586, 4.065) -> (2.1677, 4.0963)
  line L319 (2.2235, 0.584) -> (2.4076, 0.6088)
  line L320 (2.5815, 0.8087) -> (2.3791, 0.7459)
  line L321 (2.1677, 4.0963) -> (2.1903, 4.0747)
  line L322 (2.1903, 4.0747) -> (2.2068, 4.1021)
  line L323 (2.2068, 4.1021) -> (2.2233, 4.0747)
  line L324 (1.1625, 0.8028) -> (1.0713, 0.9032)
  line L325 (0.8596, 1.252) -> (0.8122, 1.3818)
  line L326 (2.0711, 3.73) -> (2.0852, 3.6373)
  line L327 (2.0852, 3.6373) -> (2.0856, 3.6278)
  line L328 (2.0856, 3.6278) -> (2.085, 3.5521)
  line L329 (2.082, 3.1979) -> (2.0814, 3.1412)
  line L330 (2.0814, 3.1412) -> (2.0766, 2.5738)
  line L331 (2.0766, 2.5738) -> (2.0762, 2.5171)
  line L332 (3.9705, 1.7978) -> (3.9705, 1.8023)
  line L333 (0.7079, 2.3168) -> (0.6747, 2.1979)
  line L334 (0.6531, 2.4375) -> (0.786, 2.4375)
  line L335 (0.786, 2.4375) -> (0.9146, 2.0279)
  line L336 (0.9146, 2.0279) -> (0.7862, 2.0276)
  line L337 (1.0838, 1.7478) -> (1.0838, 1.8021)
  line L338 (0.9444, 1.8261) -> (0.9444, 1.8201)
  line L339 (1.4813, 0.7922) -> (1.6881, 0.6799)
  line L340 (2.33, 3.7371) -> (2.3365, 3.7499)
  line L341 (2.3365, 3.7499) -> (2.3452, 3.7658)
  line L342 (2.3452, 3.7658) -> (2.355, 3.7842)
  line L343 (2.2233, 4.0747) -> (2.2459, 4.0963)
  line L344 (2.2459, 4.0963) -> (2.2549, 4.065)
  line L345 (2.2549, 4.065) -> (2.2821, 4.0792)
  line L346 (2.2162, 0.724) -> (2.1619, 0.724)
  line L347 (3, 2.0276) -> (2.9769, 2.1084)
  line L348 (0.4453, 2.4375) -> (0.4453, 2.0279)
  line L349 (0.4453, 2.0279) -> (0.3288, 2.0279)
  line L350 (3.24, 1.8261) -> (3.24, 1.8201)
  line L351 (3.24, 1.7478) -> (3.2181, 1.5849)
  line L352 (1.8288, 0.0258) -> (1.8681, 0.0189)
  line L353 (2.401, 1.3634) -> (2.3656, 1.4138)
  line L354 (2.3656, 1.4138) -> (2.3412, 1.4454)
  line L355 (2.3412, 1.4454) -> (2.3329, 1.4557)
  line L356 (1.8681, 0.0189) -> (1.8721, 0.0182)
  line L357 (1.8721, 0.0182) -> (1.8747, 0.0447)
  line L358 (0.9444, 1.8021) -> (0.9444, 1.7407)
  line L359 (0.9444, 1.7407) -> (0.9691, 1.5566)
  line L360 (2.8024, 3.327) -> (2.8024, 3.3327)
  line L361 (2.8024, 3.3327) -> (2.8024, 3.4167)
  line L362 (2.8024, 3.4167) -> (2.8024, 3.4228)
  line L363 (2.8024, 3.4228) -> (2.7975, 3.441)
  line L364 (2.7975, 3.441) -> (2.7842, 3.4608)
  line L365 (2.7842, 3.4608) -> (2.7644, 3.4742)
  line L366 (1.2813, 0.3485) -> (1.2528, 0.2712)
  line L367 (1.2528, 0.2712) -> (1.2378, 0.2492)
  line L368 (1.2378, 0.2492) -> (1.2412, 0.2471)
  line L369 (1.2412, 0.2471) -> (1.2759, 0.2272)
  line L370 (2.355, 3.7842) -> (2.3581, 3.7903)
  line L371 (2.3581, 3.7903) -> (2.3639, 3.8018)
  line L372 (2.3639, 3.8018) -> (2.3853, 3.8451)
  line L373 (1.1056, 1.5849) -> (1.0838, 1.7478)
  line L374 (2.1812, 3.1785) -> (2.1812, 3.04)
  line L375 (2.1812, 3.04) -> (2.1641, 3.04)
  line L376 (2.1641, 3.04) -> (2.1641, 3.1785)
  line L377 (1.3011, 0.9409) -> (1.4813, 0.7922)
  line L378 (2.0945, 3.0885) -> (2.2611, 3.0885)
  line L379 (1.8318, 0.1347) -> (1.8315, 0.0523)
  line L380 (0.7842, 0.6749) -> (0.7626, 0.6593)
  line L381 (1.9167, 0.6089) -> (2.1008, 0.5841)
  line L382 (2.1075, 0.724) -> (1.9446, 0.7459)
  line L383 (3.3802, 1.7407) -> (3.3802, 1.8021)
  line L384 (1.1685, 1.3824) -> (1.1056, 1.5849)
  line L385 (2.3487, 3.9768) -> (2.3273, 3.9538)
  line L386 (2.3273, 3.9538) -> (2.3514, 3.9341)
  line L387 (2.3514, 3.9341) -> (2.3251, 3.9181)
  line L388 (1.6422, 0.3729) -> (1.6672, 0.3638)
  line L389 (1.6672, 0.3638) -> (1.7354, 0.3175)
  line L390 (1.7422, 0.8087) -> (1.5591, 0.9081)
  line L391 (0.8836, 0.6825) -> (0.9862, 0.7052)
  line L392 (0.6631, 1.4297) -> (0.6239, 1.3323)
  line L393 (1.0838, 1.8261) -> (0.9444, 1.8261)
  line L394 (2.2126, 4.1664) -> (2.161, 4.1618)
  line L395 (2.161, 4.1618) -> (2.1122, 4.1445)
  line L396 (2.1122, 4.1445) -> (2.0784, 4.1236)
  line L397 (0.8317, 1.0651) -> (0.845, 1.042)
  line L398 (3.9705, 1.8081) -> (3.9692, 1.8236)
  line L399 (0.8809, 0.9398) -> (0.8776, 0.8348)
  line L400 (3.3802, 1.8081) -> (3.3802, 1.8216)
  line L401 (1.291, 0.2492) -> (1.3437, 0.3126)
  line L402 (3.4942, 1.0645) -> (3.5516, 1.1236)
  line L403 (1.2528, 0.2712) -> (1.2378, 0.2492)
  line L404 (1.8747, 0.0447) -> (1.9026, 0.1221)
  line L405 (0.4706, 1.1656) -> (0.4722, 1.1619)
  line L406 (0.4813, 1.214) -> (0.4557, 1.2069)
  line L407 (3.24, 1.8021) -> (3.24, 1.7478)
  line L408 (2.0784, 4.1236) -> (2.0686, 4.115)
  line L409 (2.0686, 4.115) -> (2.0634, 4.1109)
  line L410 (2.0634, 4.1109) -> (2.0208, 4.0609)
  line L411 (2.0096, 2.1839) -> (1.97, 2.1839)
  line L412 (1.97, 2.1839) -> (1.97, 2.0276)
  line L413 (1.157, 2.1824) -> (1.1145, 2.1221)
  line L414 (2.2089, 2.0276) -> (2.0695, 2.0276)
  line L415 (1.2532, 0.5532) -> (1.2859, 0.4534)
  line L416 (1.1642, 0.6542) -> (1.1846, 0.637)
  line L417 (1.2412, 0.2471) -> (1.2759, 0.2272)
  line L418 (3.0488, 0.2268) -> (3.0834, 0.2468)
  line L419 (0.99, 1.0119) -> (0.9192, 1.1285)
  line L420 (1.9925, 3.9145) -> (1.9938, 3.9076)
  line L421 (1.9938, 3.9076) -> (1.9956, 3.8986)
  line L422 (1.9956, 3.8986) -> (2.0101, 3.855)
  line L423 (2.3791, 0.7459) -> (2.2162, 0.724)
  line L424 (1.5352, 0.3905) -> (1.6171, 0.382)
  line L425 (2.3216, 3.7151) -> (2.3241, 3.7219)
  line L426 (2.3241, 3.7219) -> (2.3254, 3.7258)
  line L427 (2.3254, 3.7258) -> (2.33, 3.7371)
  line L428 (2.7679, 3.2772) -> (2.7859, 3.2908)
  line L429 (2.7859, 3.2908) -> (2.7979, 3.3099)
  line L430 (2.7979, 3.3099) -> (2.8024, 3.327)
  line L431 (0.5775, 1.1875) -> (0.6816, 1.1738)
  line L432 (2.307, 3.63) -> (2.307, 3.6364)
  line L433 (2.307, 3.6364) -> (2.3073, 3.6438)
  line L434 (2.3073, 3.6438) -> (2.3216, 3.7151)
  line L435 (3.24, 1.8201) -> (3.24, 1.8066)
  line L436 (1.0838, 1.8216) -> (1.0838, 1.8261)
  line L437 (2.9242, 1.0398) -> (2.7647, 0.9081)
  line L438 (2.8925, 0.3688) -> (2.9811, 0.3122)
  line L439 (2.9811, 0.3122) -> (3.0337, 0.2489)
  line L440 (3.0337, 0.2489) -> (3.0453, 0.2249)
  line L441 (3.0453, 0.2249) -> (3.0488, 0.2268)
  line L442 (2.0892, 3.1875) -> (2.2142, 3.1875)
  line L443 (0.9444, 1.8066) -> (0.9444, 1.8021)
  line L444 (3.24, 1.8066) -> (3.24, 1.8021)
  line L445 (3.9705, 1.7778) -> (3.9705, 1.784)
  line L446 (1.6672, 0.3638) -> (1.7354, 0.3175)
  line L447 (2.1081, 4.0203) -> (2.1009, 4.0521)
  line L448 (2.29, 2.7214) -> (2.299, 3.1979)
  line L449 (2.2821, 4.0792) -> (2.283, 4.0464)
  line L450 (2.283, 4.0464) -> (2.3127, 4.0521)
  line L451 (2.3127, 4.0521) -> (2.3055, 4.0203)
  line L452 (2.0101, 3.855) -> (2.0312, 3.8142)
  line L453 (2.0312, 3.8142) -> (2.0364, 3.8065)
  line L454 (2.1009, 4.0521) -> (2.1305, 4.0464)
  line L455 (2.0892, 2.8333) -> (2.0892, 3.1875)
  line L456 (0.7862, 2.0276) -> (0.7631, 2.1084)
  line L457 (0.9691, 1.5566) -> (1.04, 1.3281)
  line L458 (1.04, 1.3281) -> (1.1523, 1.1212)
  line L459 (3.9194, 1.8261) -> (3.5751, 1.8261)
  line L460 (3.965, 1.8253) -> (3.9235, 1.8257)
  line L461 (2.1619, 0.724) -> (2.1075, 0.724)
  line L462 (3.0234, 0.9408) -> (3.1722, 1.1211)
  line L463 (1.5632, 3.4167) -> (1.5632, 3.3333)
  line L464 (1.5632, 3.3333) -> (1.5631, 3.3276)
  line L465 (2.085, 3.5521) -> (2.3058, 3.5521)
  line L466 (2.3058, 3.5521) -> (2.307, 3.6107)
  line L467 (2.307, 3.6107) -> (2.307, 3.63)
  line L468 (0.9444, 1.8201) -> (0.9444, 1.8066)
  line L469 (2.0398, 3.8017) -> (2.0659, 3.7483)
  line L470 (2.0659, 3.7483) -> (2.0676, 3.7425)
  line L471 (2.0676, 3.7425) -> (2.0676, 3.7416)
  line L472 (3.1553, 1.3824) -> (3.0559, 1.1993)
  line L473 (0.9955, 2.4375) -> (1.114, 2.4375)
  line L474 (1.114, 2.4375) -> (1.114, 2.2681)
  line L475 (3.0834, 0.2468) -> (3.087, 0.2489)
  line L476 (3.087, 0.2489) -> (3.0719, 0.2709)
  line L477 (3.0719, 0.2709) -> (3.0435, 0.3482)
  line L478 (1.4324, 0.369) -> (1.5352, 0.3905)
  line L479 (1.5352, 0.3905) -> (1.6171, 0.382)
  line L480 (1.6171, 0.382) -> (1.6422, 0.3729)
  line L481 (2.2142, 3.1875) -> (2.2142, 2.8333)
  line L482 (2.0676, 3.7416) -> (2.0685, 3.7393)
  line L483 (2.0685, 3.7393) -> (2.0686, 3.739)
  line L484 (2.0686, 3.739) -> (2.0711, 3.73)
  line L485 (0.7907, 0.6255) -> (0.7933, 0.6225)
  line L486 (3.7698, 1.7171) -> (3.8629, 1.7657)
  line L487 (1.6881, 0.6799) -> (1.9167, 0.6089)
  line L488 (2.0208, 4.0609) -> (2.0175, 4.0551)
  line L489 (2.0175, 4.0551) -> (2.0147, 4.0501)
  line L490 (2.0147, 4.0501) -> (1.9948, 3.9966)
  line L491 (3.9235, 1.8257) -> (3.9194, 1.8261)
  line L492 (0.6287, 2.0276) -> (0.5267, 2.0276)
  line L493 (2.4006, 3.8841) -> (2.4038, 3.8937)
  line L494 (2.4038, 3.8937) -> (2.4123, 3.9435)
  line L495 (2.4123, 3.9435) -> (2.4109, 3.9939)
  line L496 (2.4664, 1.2329) -> (2.4603, 1.25)
  line L497 (2.4603, 1.25) -> (2.4607, 1.2504)
  line L498 (0.741, 2.1979) -> (0.7079, 2.3168)
  line L499 (0.6533, 2.1084) -> (0.6287, 2.0276)
  line L500 (0.5267, 2.0276) -> (0.6531, 2.4375)
  line L501 (0.2531, 2.0276) -> (0.1726, 2.0276)
  line L502 (0.1726, 2.0276) -> (0.0938, 2.3204)
  line L503 (0.0938, 2.3204) -> (0.0938, 2.0276)
  line L504 (3.3802, 1.8021) -> (3.3802, 1.8081)
  line L505 (3.3802, 1.7407) -> (3.3802, 1.8021)
  line L506 (2.4665, 1.0268) -> (2.4693, 1.037)
  line L507 (2.4693, 1.037) -> (2.4739, 1.0546)
  line L508 (2.4739, 1.0546) -> (2.4808, 1.1442)
  line L509 (2.4808, 1.1442) -> (2.4664, 1.2329)
  line L510 (2.6594, 2.4375) -> (2.6594, 2.0279)
  line L511 (3.4656, 2.1809) -> (3.3321, 2.1809)
  line L512 (3.2097, 2.0276) -> (3.2097, 2.4375)
  line L513 (2.8886, 2.1979) -> (2.9548, 2.1979)
  line L514 (1.0838, 1.8021) -> (1.0838, 1.8081)
  line L515 (2.0945, 2.5781) -> (2.0945, 3.0885)
  line L516 (2.952, 0.6302) -> (2.8355, 0.5595)
  line L517 (0.6264, 1.6395) -> (0.6599, 1.5643)
  line L518 (2.0059, 3.2708) -> (2.1778, 3.2708)
  line L519 (2.1778, 3.2708) -> (2.1778, 3.4167)
  line L520 (2.1778, 3.4167) -> (2.1882, 3.4167)
  line L521 (2.5821, 0.4524) -> (2.4467, 0.4176)
  line L522 (0.7486, 1.8021) -> (0.7486, 1.8081)
  line L523 (3.24, 1.7478) -> (3.2181, 1.5849)
  line L524 (0.7486, 1.766) -> (0.7486, 1.8021)
  line L525 (1.0838, 1.8081) -> (1.0838, 1.8216)
  line L526 (3.2181, 1.5849) -> (3.1553, 1.3824)
  line L527 (0.3556, 1.7787) -> (0.3822, 1.7807)
  line L528 (0.7486, 1.8216) -> (0.7486, 1.8261)
  line L529 (3.5751, 1.8021) -> (3.5751, 1.766)
  line L530 (0.3927, 1.8261) -> (0.386, 1.8261)
  line L531 (2.2611, 3.0885) -> (2.2611, 2.5781)
  line L532 (0.5528, 1.2549) -> (0.4813, 1.214)
  line L533 (3.5463, 1.5173) -> (3.5115, 1.3818)
  line L534 (2.7455, 3.4167) -> (2.7455, 3.2708)
  line L535 (2.7455, 3.2708) -> (2.7511, 3.2714)
  line L536 (2.7511, 3.2714) -> (2.7679, 3.2772)
  line L537 (0.3556, 1.8201) -> (0.3556, 1.8066)
  line L538 (3.0608, 0.7116) -> (2.952, 0.6302)
  line L539 (2.5788, 3.2708) -> (2.7351, 3.2708)
  line L540 (2.7351, 3.2708) -> (2.7351, 3.4167)
  line L541 (2.7351, 3.4167) -> (2.7455, 3.4167)
  line L542 (2.057, 0.8298) -> (2.0562, 0.8322)
  line L543 (2.0562, 0.8322) -> (2.0562, 0.8324)
  line L544 (2.0562, 0.8324) -> (2.0049, 1.0857)
  line L545 (2.0049, 1.0857) -> (2.0039, 1.0902)
  line L546 (1.8771, 0.4176) -> (1.7416, 0.4524)
  line L547 (2.6827, 0.3728) -> (2.7077, 0.3819)
  line L548 (2.7077, 0.3819) -> (2.7896, 0.3903)
  line L549 (2.7896, 0.3903) -> (2.8925, 0.3688)
  line L550 (2.1882, 3.4167) -> (2.1882, 3.2708)
  line L551 (2.1882, 3.2708) -> (2.3705, 3.2708)
  line L552 (2.3705, 3.2708) -> (2.3705, 3.3438)
  line L553 (3.7698, 1.7171) -> (3.8629, 1.7657)
  line L554 (3.8629, 1.7657) -> (3.944, 1.7798)
  line L555 (0.7486, 1.8261) -> (0.3927, 1.8261)
  line L556 (3.5678, 1.6576) -> (3.5463, 1.5173)
  line L557 (0.6599, 1.5643) -> (0.6646, 1.5381)
  line L558 (0.9444, 1.8261) -> (0.9444, 1.8201)
  line L559 (2.2989, 1.507) -> (2.2947, 1.5143)
  line L560 (2.2946, 1.5143) -> (2.2828, 1.5366)
  line L561 (2.2828, 1.5366) -> (2.2728, 1.5597)
  line L562 (0.8596, 1.252) -> (0.8122, 1.3818)
  line L563 (0.457, 1.2031) -> (0.4706, 1.1656)
  line L564 (2.2649, 1.6268) -> (2.2655, 1.6521)
  line L565 (2.2655, 1.6521) -> (2.2713, 1.9044)
  line L566 (2.2713, 1.9044) -> (2.2719, 1.9296)
  line L567 (1.9786, 0.8878) -> (2.0213, 0.8522)
  line L568 (2.0213, 0.8522) -> (2.0258, 0.849)
  line L569 (2.0258, 0.849) -> (2.0284, 0.8471)
  line L570 (2.0284, 0.8471) -> (2.0545, 0.8309)
  line L571 (2.8355, 0.5595) -> (2.712, 0.4999)
  line L572 (3.5751, 1.766) -> (3.5678, 1.6576)
  line L573 (3.1553, 1.3824) -> (3.0559, 1.1993)
  line L574 (3.5115, 1.3818) -> (3.464, 1.252)
  line L575 (2.0945, 3.0885) -> (2.2611, 3.0885)
  line L576 (2.712, 0.4999) -> (2.5821, 0.4524)
  line L577 (3.1722, 1.1211) -> (3.2844, 1.328)
  line L578 (0.386, 1.8261) -> (0.371, 1.8261)
  line L579 (3.5678, 1.6576) -> (3.5463, 1.5173)
  line L580 (1.6309, 3.4167) -> (1.6309, 3.2708)
  line L581 (1.6309, 3.2708) -> (1.808, 3.2708)
  line L582 (2.2856, 2.5341) -> (2.2896, 2.7044)
  line L583 (2.0545, 0.8309) -> (2.0571, 0.8295)
  line L584 (2.0571, 0.8295) -> (2.057, 0.8298)
  line L585 (2.5245, 0.2349) -> (2.5894, 0.3175)
  line L586 (2.5894, 0.3175) -> (2.6576, 0.3637)
  line L587 (2.6576, 0.3637) -> (2.6827, 0.3728)
  line L588 (0.5564, 1.7179) -> (0.6264, 1.6395)
  line L589 (0.9444, 1.8201) -> (0.9444, 1.8066)
  line L590 (3.5751, 1.8261) -> (3.5751, 1.8201)
  line L591 (2.1258, 0.3888) -> (2.0174, 0.3962)
  line L592 (0.7559, 1.6576) -> (0.7486, 1.766)
  line L593 (2.1258, 0.3888) -> (2.0174, 0.3962)
  line L594 (1.0838, 1.8261) -> (0.9444, 1.8261)
  line L595 (2.5815, 0.8087) -> (2.3791, 0.7459)
  line L596 (0.7486, 1.8021) -> (0.7486, 1.8081)
  line L597 (1.1625, 0.8028) -> (1.0713, 0.9032)
  line L598 (1.0713, 0.9032) -> (0.99, 1.0119)
  line L599 (1.04, 1.3281) -> (1.1523, 1.1212)
  line L600 (3.5751, 1.8021) -> (3.5751, 1.766)
  line L601 (0.4633, 1.7665) -> (0.5564, 1.7179)
  line L602 (1.4882, 0.5595) -> (1.3717, 0.6302)
  line L603 (2.4928, 0.1347) -> (2.5245, 0.2349)
  line L604 (0.3556, 1.8261) -> (0.3556, 1.8201)
  line L605 (2.0649, 3.9768) -> (2.0929, 3.9887)
  line L606 (1.9167, 0.6089) -> (2.1008, 0.5841)
  line L607 (3.3802, 1.8216) -> (3.3802, 1.8261)
  line L608 (1.8771, 0.4176) -> (1.7416, 0.4524)
  line L609 (2.2162, 0.724) -> (2.1619, 0.724)
  line L610 (3.2523, 0.9032) -> (3.1611, 0.8028)
  line L611 (0.3822, 1.7807) -> (0.4633, 1.7665)
  line L612 (2.3064, 0.3962) -> (2.198, 0.3888)
  line L613 (3.1611, 0.8028) -> (3.0608, 0.7116)
  line L614 (0.7486, 1.766) -> (0.7486, 1.8021)
  line L615 (3.0559, 1.1993) -> (2.9242, 1.0398)
  line L616 (3.8701, 1.2062) -> (3.8445, 1.2134)
  line L617 (3.8445, 1.2134) -> (3.773, 1.2543)
  line L618 (1.5591, 0.9081) -> (1.3995, 1.0398)
  line L619 (2.2696, 3.8332) -> (2.2646, 3.8011)
  line L620 (2.2646, 3.8011) -> (2.2394, 3.8191)
  line L621 (2.2394, 3.8191) -> (2.2266, 3.7895)
  line L622 (0.6239, 1.3323) -> (0.5528, 1.2549)
  line L623 (1.3011, 0.9409) -> (1.4813, 0.7922)
  line L624 (0.371, 1.8261) -> (0.366, 1.8261)
  line L625 (0.7486, 1.8261) -> (0.3927, 1.8261)
  line L626 (0.4722, 1.1619) -> (0.4964, 1.1729)
  line L627 (3.9194, 1.8261) -> (3.5751, 1.8261)
  line L628 (3.9705, 1.7978) -> (3.9705, 1.8023)
  line L629 (3.9705, 1.8023) -> (3.9705, 1.8081)
  line L630 (0.7743, 1.1242) -> (0.8317, 1.0651)
  line L631 (1.9035, 0.975) -> (1.9338, 0.9332)
  line L632 (1.9338, 0.9332) -> (1.9675, 0.8985)
  line L633 (1.9675, 0.8985) -> (1.9747, 0.8917)
  line L634 (1.9747, 0.8917) -> (1.9786, 0.8878)
  line L635 (1.7153, 2.1926) -> (1.5659, 2.1926)
  line L636 (1.5659, 2.1926) -> (1.5659, 2.125)
  line L637 (1.5659, 2.125) -> (1.7507, 2.125)
  line L638 (3.9235, 1.8257) -> (3.9194, 1.8261)
  line L639 (0.8122, 1.3818) -> (0.7773, 1.5173)
  line L640 (0.7486, 1.8081) -> (0.7486, 1.8216)
  line L641 (3.5751, 1.766) -> (3.5678, 1.6576)
  line L642 (1.9955, 3.2708) -> (1.9955, 3.3438)
  line L643 (1.9955, 3.3438) -> (2.0059, 3.3438)
  line L644 (2.0059, 3.3438) -> (2.0059, 3.2708)
  line L645 (2.1619, 0.3888) -> (2.1258, 0.3888)
  line L646 (0.7486, 1.8081) -> (0.7486, 1.8216)
  line L647 (3.24, 1.8021) -> (3.24, 1.7478)
  line L648 (0.6646, 1.5381) -> (0.6691, 1.5119)
  line L649 (3.5751, 1.8201) -> (3.5751, 1.8066)
  line L650 (2.3705, 3.3438) -> (2.3809, 3.3438)
  line L651 (2.3809, 3.3438) -> (2.3809, 3.2708)
  line L652 (2.3809, 3.2708) -> (2.5684, 3.2708)
  line L653 (3.3802, 1.8261) -> (3.24, 1.8261)
  line L654 (0.3556, 1.8021) -> (0.3556, 1.7962)
  line L655 (1.808, 3.2708) -> (1.808, 3.3438)